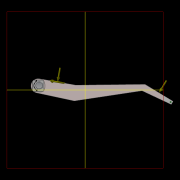
# Autodesk Inventor part: forearm
Saved by Autodesk Inventor 2020 (Build 240168000, 168)
## iProperties
Created: 2020-03-28
Part Number: forearm
Material: Generic
Document SubType Name: Modeling
Designer: valer
Density: 1 g/cm^3
Appearance: Default
Author: valer
Autodesk Inventor part; units mm, degrees
ref_plane "YZ Plane" through (0, 0, 0) normal (1, 0, 0) x (0, 1, 0)
ref_plane "XZ Plane" through (0, 0, 0) normal (0, 1, 0) x (-1, 0, 0)
ref_plane "XY Plane" through (0, 0, 0) normal (0, 0, 1) x (1, 0, 0)
sketch "Sketch1" plane through (0, 0, 0) normal (0, 0, 1) x (1, 0, 0)
  line L0 (131.4017, -33.1581) -> (234.4053, -26.2304) construction
  line L1 (375.2105, -13.3271) -> (477.233, -67.9218) construction
  line L2 (380.4679, -2.1311) -> (480.5131, -62.4845)
  line L3 (480.5131, -62.4845) -> (473.953, -73.359)
  line L4 (369.9531, -24.5231) -> (473.953, -73.359)
  line L5 (380.4679, -2.1311) -> (369.9531, -24.5231) construction
  line L6 (128.7595, -60.7752) -> (134.1036, -4.9164) construction
  line L7 (128.7595, -60.7752) -> (-5.3656, -32.0813)
  circle A0 centre (-0.0519, -7.2434) radius 25.4
  line L8 (134.1036, -4.9164) -> (4.3231, 17.777)
  line L9 (131.4017, -33.1581) -> (-0.0519, -7.2434) construction
  line L10 (265.3565, -22.0515) -> (375.2105, -13.3271) construction
  line L11 (134.1036, -4.9164) -> (380.4679, -2.1311)
  line L12 (128.7595, -60.7752) -> (369.9531, -24.5231)
  circle A1 centre (471.6268, -64.9218) radius 3.175
  circle A2 centre (-0.0519, -7.2434) radius 3.175
  point P0 (0, 0)
  dimension "d4" = 148
  dimension "d5" = 50.8
  dimension "d6" = 24.7379
  dimension "d7" = 165
  dimension "d8" = 4.7
  dimension "d9" = 3.2
  dimension "d10" = 137.16
  dimension "d11" = 246.38
  dimension "d12" = 116.84
  dimension "d13" = 12.7
  dimension "d14" = 6.35
  dimension "d15" = 6.35
  dimension "d16" = 6.35
  constraints: 26 end point, 3 centre point, 2 midpoint, 2 perpendicular, 2 point on circle, 2 point on line, 2 tangent, 1 coincident, 2 other
  measures "d4" angle of L1 L0
  measures "d5" diameter of A0
  measures "d6" distance of L2.start L4.start
  measures "d7" angle of L0 L9
  measures "d8" angle of L12 L0
  measures "d9" angle of L11 L0
  measures "d10" distance of L6.start L7.end
  measures "d11" distance of L6.end L2.start
  measures "d12" distance of L2.start L2.end
  measures "d13" distance of L2.end L3.end
  measures "d14" diameter of A1
  measures "d15" distance from line of L3 A1.centre
  measures "d16" diameter of A2
extrude "Extrusion1" add sketch "Sketch1" along normal mid plane 20.32 contours L2 L3 L4 L12 L7 A0 L8 L11
extrude "Extrusion2" add sketch "Sketch1" along normal mid plane 38.1 contours A0
body "Solid1"
